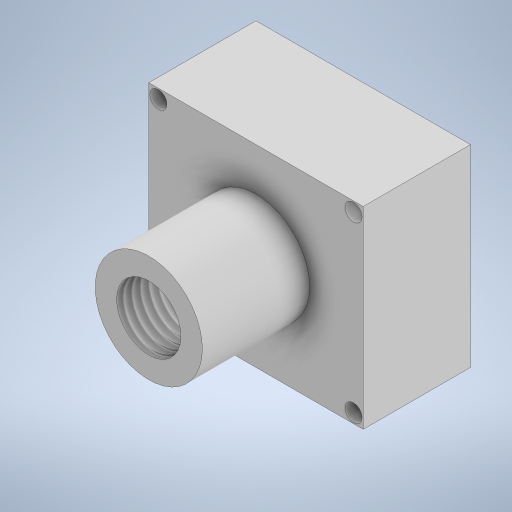
# Autodesk Inventor part: Práctica #1 Conociendo inventor
Saved by Autodesk Inventor 2024 (Build 280153000, 153)
## iProperties
Created: 2024-02-06
Part Number: Práctica #1 Conociendo inventor
Material: Generic
Document SubType Name: Sheet Metal
Designer: mater
Density: 1 g/cm^3
Sheet Metal Rule: Default
Appearance: Default
Author: mater
Autodesk Inventor part; units mm, degrees
ref_plane "YZ Plane" through (0, 0, 0) normal (1, 0, 0) x (0, 1, 0)
ref_plane "XZ Plane" through (0, 0, 0) normal (0, 1, 0) x (-1, 0, 0)
ref_plane "XY Plane" through (0, 0, 0) normal (0, 0, 1) x (1, 0, 0)
sketch "Sketch1" plane through (0, 0, 0) normal (0, 0, 1) x (1, 0, 0)
  line L0 (-50, 45) -> (50, 45)
  line L1 (50, 45) -> (50, -45)
  line L2 (50, -45) -> (-50, -45)
  line L3 (-50, -45) -> (-50, 45)
  line L4 (-50, 45) -> (50, -45) construction
  line L5 (50, 45) -> (-50, -45) construction
  point P0 (0, 0)
  constraints: 12 end point, 2 midpoint, 2 parallel, 1 horizontal, 1 perpendicular
extrude "Extrusion1" add sketch "Sketch1" along normal blind 50
sketch "Sketch5" plane through (0, 0, 50) normal (0, 0, 1) x (1, 0, 0)
  point P0 (0, 0)
sketch "Sketch6" plane through (0, 0, 50) normal (0, 0, 1) x (1, 0, 0)
  line L0 (50, 45) -> (41, 45)
  circle A0 centre (45.5, 40.5) radius 4
  point P0 (0, 0)
  constraints: 2 end point, 1 centre point, 1 horizontal
extrude "Extrusion3" cut sketch "Sketch6" against normal blind 50
sketch "Sketch7" plane through (0, 0, 50) normal (0, 0, 1) x (1, 0, 0)
  circle A0 centre (-45.5, -40.5) radius 4
  circle A1 centre (45.5, -40.5) radius 4
  circle A2 centre (-45.5, 40.5) radius 4
  point P0 (0, 0)
  point P1 (-50, -45)
  point P2 (50, -45)
  constraints: 3 centre point
extrude "Extrusion4" cut sketch "Sketch7" against normal blind 50 contours A2
sketch "Sketch8" plane through (0, 0, 50) normal (0, 0, 1) x (1, 0, 0)
  line L0 (-50, -45) -> (50, -45) projected
  line L1 (-50, -45) -> (-41, -45)
  line L2 (-41, -45) -> (-41, -36)
  line L3 (-41, -36) -> (-50, -36)
  line L4 (-50, -36) -> (-50, -45)
  line L5 (50, -45) -> (50, 45) projected
  line L6 (50, -45) -> (41, -45)
  line L7 (41, -45) -> (41, -36)
  line L8 (41, -36) -> (50, -36)
  line L9 (50, -36) -> (50, -45)
  circle A0 centre (45.5, -40.5) radius 4
  circle A1 centre (-45.5, -40.5) radius 4
  point P0 (0, 0)
  dimension "d45" = 9
  dimension "d46" = 9
  dimension "d47" = 8
  dimension "d48" = 8
  constraints: 16 end point, 4 parallel, 2 centre point, 2 horizontal, 2 perpendicular
  measures "d45" distance of L7.end L8.end
  measures "d46" distance of L6.end L7.end
  measures "d47" diameter of A0
  measures "d48" diameter of A1
extrude "Extrusion5" cut sketch "Sketch8" against normal blind 50 contours A0
sketch "Sketch9" plane through (0, 0, 50) normal (0, 0, 1) x (1, 0, 0)
  circle A0 centre (0, 0) radius 15
  constraints: 1 centre point, 1 coincident
sketch "Sketch10" plane through (0, 0, 50) normal (0, 0, 1) x (1, 0, 0)
  line L0 (-50, 45) -> (-50, -45) projected
  line L1 (-50, -45) -> (-41, -45)
  line L2 (-41, -45) -> (-41, -36)
  line L3 (-41, -36) -> (-50, -36)
  line L4 (-50, -36) -> (-50, -45)
  circle A0 centre (-45.5, -40.5) radius 4
  point P0 (0, 0)
  dimension "d51" = 9
  dimension "d52" = 9
  dimension "d53" = 8
  constraints: 8 end point, 2 parallel, 1 centre point, 1 horizontal, 1 perpendicular
  measures "d51" distance of L3.end L2.end
  measures "d52" distance of L2.end L1.end
  measures "d53" diameter of A0
extrude "Extrusion6" cut sketch "Sketch10" against normal blind 50 contours A0
sketch "Sketch11" plane through (0, 0, 50) normal (0, 0, 1) x (1, 0, 0)
  circle A0 centre (0, 0) radius 25
  dimension "d58" = 50
  constraints: 1 centre point, 1 coincident
  measures "d58" diameter of A0
extrude "Extrusion7" add sketch "Sketch11" along normal blind 50
sketch "Sketch12" plane through (0, 0, 100) normal (0, 0, 1) x (1, 0, 0)
  circle A0 centre (0, 0) radius 15
  dimension "d61" = 30
  constraints: 1 centre point, 1 coincident
  measures "d61" diameter of A0
extrude "Extrusion8" cut sketch "Sketch12" against normal blind 30
thread "Thread2" size "M50x4" class "6H" standard "ANSI Metric M Profile" length 25.616
equation "\"BendRadius\" = Thickness"
equation "\"BendReliefWidth\" = Thickness"
equation "\"BendReliefDepth\" = 0.5 * Thickness"
equation "\"CornerReliefSize\" = 4 * Thickness"
equation "\"MinimumRemnant\" = 2 * Thickness"
equation "\"TransitionRadius\" = BendRadius"
equation "\"JacobiRadiusSize\" = BendRadius"
equation "\"GapSize\" = Thickness"
equation "\"Thickness\" = 3.048"
body "Solid1"
